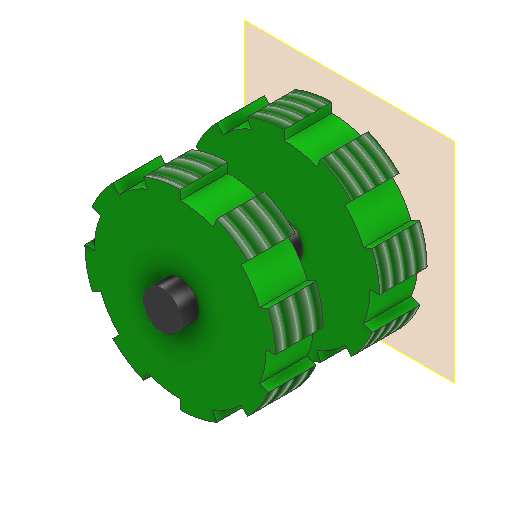
# Autodesk Inventor part: Coletor - Hand
Saved by Autodesk Inventor 2025.3 (Build 293356000, 356)
## iProperties
Created: 2026-05-13
Part Number: Coletor - Hand
Material: Genérico
Document SubType Name: Modeling
Designer: djair.oliveira
Density: 1 g/cm^3
Appearance: Padrão
Author: djair.oliveira
Autodesk Inventor part; units mm, degrees
ref_plane "YZ Plane" through (0, 0, 0) normal (1, 0, 0) x (0, 1, 0)
ref_plane "XZ Plane" through (0, 0, 0) normal (0, 1, 0) x (-1, 0, 0)
sketch "Esboço1" plane through (0, 0, 0) normal (1, 0, 0) x (0, 1, 0)
  line L0 (0, 0) -> (0, 100)
  line L1 (0, 100) -> (10, 100)
  line L2 (10, 100) -> (10, 90.4)
  line L3 (10, 90.4) -> (50.8, 90.4)
  line L4 (50.8, 90.4) -> (50.8, 65)
  line L5 (50.8, 65) -> (10, 65)
  line L6 (10, 65) -> (10, 35)
  line L7 (10, 35) -> (50.8, 35)
  line L8 (50.8, 35) -> (50.8, 9.6)
  line L9 (50.8, 9.6) -> (10, 9.6)
  line L10 (10, 9.6) -> (10, 0)
  line L11 (10, 0) -> (0, 0)
  line L12 (0, 50) -> (10, 50)
  dimension "d0" = 10
  dimension "d1" = 100
  dimension "d2" = 25.4
  dimension "d3" = 25.4
  dimension "d4" = 15
  dimension "d5" = 15
  dimension "d6" = 50.8
  constraints: 26 end point, 8 perpendicular, 6 point on line, 2 midpoint, 1 horizontal, 1 vertical
  measures "d0" distance of L10.end L0.start
  measures "d1" distance of L0.start L0.end
  measures "d2" distance of L3.end L4.end
  measures "d3" distance of L7.end L8.end
  measures "d4" distance between parallel lines of L5 L12
  measures "d5" distance between parallel lines of L12 L7
  measures "d6" distance between parallel lines of L0 L4
revolve "Revolução1" add sketch "Esboço1" angle 360 about axis through (0, 0, 0) along (0, 0, 1)
thread "Rosca1" size "M1060x8" class "6g" standard "ANSI Metric M Profile" full length
thread "Rosca2" size "M105x6" class "6g" standard "ANSI Metric M Profile" full length
sketch "Esboço4" plane through (0, 0, 90.4) normal (0, 0, 1) x (1, 0, 0)
  circle A0 centre (0, 0) radius 10 projected
  circle A1 centre (0, 0) radius 50.8 projected
  line L0 (0, 0) -> (0, 50.8)
  line L1 (0, 0) -> (0, -50.8)
  line L2 (0, 0) -> (50.8, 0)
  line L3 (0, 0) -> (-50.8, 0)
  line L4 (0, 0) -> (-35.921, 35.921)
  line L5 (0, 0) -> (-19.4403, 46.9331)
  line L6 (0, 0) -> (-46.9331, 19.4403)
  line L7 (0, 0) -> (35.921, 35.921)
  line L8 (0, 0) -> (19.4403, 46.9331)
  line L9 (0, 0) -> (46.9331, 19.4403)
  line L10 (0, 0) -> (-35.921, -35.921)
  line L11 (0, 0) -> (-19.4403, -46.9331)
  line L12 (0, 0) -> (-46.9331, -19.4403)
  line L13 (0, 0) -> (19.4403, -46.9331)
  line L14 (0, 0) -> (35.921, -35.921)
  line L15 (0, 0) -> (46.9331, -19.4403)
  circle A2 centre (0, 0) radius 45.8
  point P0 (-5, 45.5263)
  point P1 (-45.8, 0)
  point P2 (0, -45.8)
  point P3 (45.8, 0)
  point P4 (0, 45.8)
  point P5 (-42.3137, -17.5269)
  point P6 (17.5269, -42.3137)
  point P7 (42.3137, 17.5269)
  point P8 (-17.5269, 42.3137)
  point P9 (17.5269, 42.3137)
  point P10 (42.3137, -17.5269)
  point P11 (32.3855, 32.3855)
  point P12 (32.3855, -32.3855)
  point P13 (-32.3855, 32.3855)
  point P14 (-42.3137, 17.5269)
  point P15 (-32.3855, -32.3855)
  point P16 (-17.5269, -42.3137)
  dimension "d21" = 45
  dimension "d22" = 22.5
  dimension "d23" = 22.5
  constraints: 32 end point, 9 symmetric about line, 1 coincident, 1 perpendicular, 1 point on line, 1 vertical, 11 other
  measures "d21" angle of L3 L4
  measures "d22" angle of L6 L4
  measures "d23" angle of L0 L5
extrude "Extrusão3" cut sketch "Esboço4" against normal up to surface (80.8 mm away) contours L2 A1 L15 A2 | A2 L7 A1 L9 | L14 A1 L13 A2 | L0 A1 L8 A2 | L1 A1 L11 A2 | L3 A1 L6 A2 | L4 A1 L5 A2 | L10 A1 L12 A2
equation "\"d3\" = d2"
equation "\"d5\" = d4"
equation "\"d22\" = 0.5 * d21"
equation "\"d23\" = d22"
